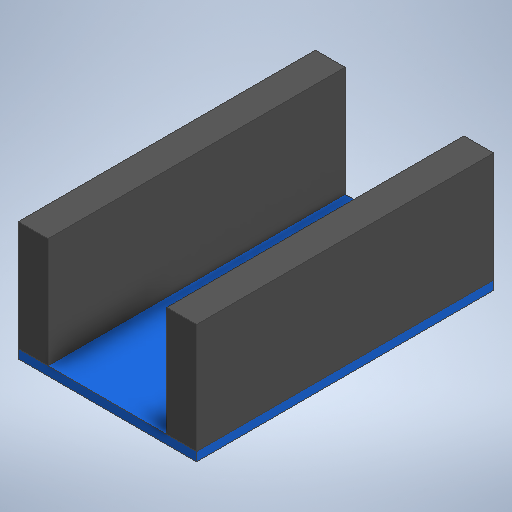
# Autodesk Inventor part: voltageconverter
Saved by Autodesk Inventor 2025 (Build 290162000, 162)
## iProperties
Created: 2025-05-12
Part Number: voltageconverter
Material: Generic
Document SubType Name: Modeling
Designer: ethan
Density: 1 g/cm^3
Appearance: Default
Author: ethan
Autodesk Inventor part; units mm, degrees
ref_plane "YZ Plane" through (0, 0, 0) normal (1, 0, 0) x (0, 1, 0)
ref_plane "XZ Plane" through (0, 0, 0) normal (0, 1, 0) x (-1, 0, 0)
ref_plane "XY Plane" through (0, 0, 0) normal (0, 0, 1) x (1, 0, 0)
sketch "Sketch1" plane through (0, 0, 0) normal (0, 1, 0) x (-1, 0, 0)
  line L0 (-7.62, 12.7) -> (7.62, 12.7)
  line L1 (7.62, 12.7) -> (7.62, -12.7)
  line L2 (7.62, -12.7) -> (-7.62, -12.7)
  line L3 (-7.62, -12.7) -> (-7.62, 12.7)
  line L4 (-7.62, 12.7) -> (7.62, -12.7) construction
  line L5 (7.62, 12.7) -> (-7.62, -12.7) construction
  point P0 (0, 0)
  dimension "d0" = 15.24
  dimension "d1" = 25.4
  constraints: 12 end point, 2 midpoint, 2 parallel, 1 horizontal, 1 perpendicular
  measures "d0" distance of L1.end L2.end
  measures "d1" distance of L0.end L1.end
extrude "Extrusion1" add sketch "Sketch1" along normal blind 0.762
sketch "Sketch3" plane through (0, 0.762, 0) normal (0, 1, 0) x (1, 0, 0)
  line L0 (7.62, 12.7) -> (-7.62, 12.7) projected
  line L1 (-7.62, 12.7) -> (-7.62, -12.7) projected
  line L2 (-7.62, -12.7) -> (7.62, -12.7) projected
  line L3 (7.62, -12.7) -> (7.62, 12.7) projected
  line L4 (-7.62, -12.7) -> (-5.08, -12.7)
  line L5 (-5.08, -12.7) -> (-5.08, 12.7)
  line L6 (-5.08, 12.7) -> (-7.62, 12.7)
  line L7 (-7.62, 12.7) -> (-7.62, -12.7)
  line L8 (7.62, 12.7) -> (5.08, 12.7)
  line L9 (5.08, 12.7) -> (5.08, -12.7)
  line L10 (5.08, -12.7) -> (7.62, -12.7)
  line L11 (7.62, -12.7) -> (7.62, 12.7)
  point P0 (0, 0)
  dimension "d7" = 2.54
  dimension "d8" = 2.54
  constraints: 16 end point, 4 parallel, 2 horizontal, 2 perpendicular, 2 point on line
  measures "d7" distance of L6.end L5.end
  measures "d8" distance of L10.end L9.end
extrude "Extrusion3" add sketch "Sketch3" along normal blind 9.398 separate body contours L3 L2 L9 L0 | L5 L2 L1 L0
body "Solid1"
body "Solid2"
